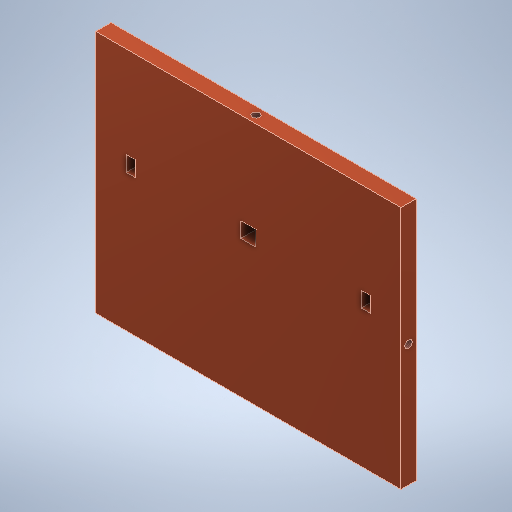
# Autodesk Inventor part: chassis arriere
Saved by Autodesk Inventor 2026.2 (Build 302298010, 298A)
## iProperties
Created: 2026-03-16
Part Number: chassis arriere
Material: Générique
Document SubType Name: Modeling
Designer: genon
Density: 1 g/cm^3
Appearance: Cuivre - Satiné
Author: genon
Autodesk Inventor part; units mm, degrees
ref_plane "YZ Plane" through (0, 0, 0) normal (1, 0, 0) x (0, 1, 0)
ref_plane "XZ Plane" through (0, 0, 0) normal (0, 1, 0) x (-1, 0, 0)
ref_plane "XY Plane" through (0, 0, 0) normal (0, 0, 1) x (1, 0, 0)
sketch "Esquisse1" plane through (0, 0, 0) normal (0, 0, 1) x (1, 0, 0)
  line L0 (0, 0) -> (100, 0)
  line L1 (100, 0) -> (100, 80)
  line L2 (100, 80) -> (0, 80)
  line L3 (0, 80) -> (0, 0)
  dimension "d0" = 100
  dimension "d1" = 80
  constraints: 8 end point, 2 parallel, 1 horizontal, 1 perpendicular
  measures "d0" distance of L2.end L1.end
  measures "d1" distance of L1.end L0.end
extrude "Extrusion1" add sketch "Esquisse1" against normal blind 5
sketch "Esquisse3" plane through (100, 0, 0) normal (1, 0, 0) x (0, 0, -1)
  line L0 (0, 0) -> (0, 80) projected
  line L1 (0, 80) -> (0, 40)
  line L2 (0, 40) -> (2.5, 40)
  line L3 (0, 40) -> (2.5, 40) construction
  line L4 (0, 0) -> (2.5, 0)
  dimension "d4" = 40
  dimension "d5" = 2.5
  dimension "d6" = 0
  constraints: 8 end point, 3 horizontal, 1 coincident, 1 collinear, 1 midpoint
  measures "d4" distance of L0.end L1.end
  measures "d5" distance of L1.end L2.end
  measures "d6" distance between parallel lines of L2 L3
hole "Perçage1" at (100, 40, -2.5) direction (-1, 0, 0) diameter 2.459 depth 8.8 tip angle 118 thread size "M3x0.5" class "6H" standard "ISO Metric profile"
sketch "Esquisse4" plane through (0, 0, 0) normal (-1, 0, 0) x (0, 0, 1)
  line L0 (0, 0) -> (-5, 0) projected
  line L1 (0, 0) -> (0, 80) projected
  line L2 (0, 80) -> (-2.5, 80)
  line L3 (-2.5, 80) -> (-2.5, 40)
  dimension "d17" = 40
  dimension "d18" = 90
  dimension "d52" = 2.5
  constraints: 4 end point, 1 coincident, 1 horizontal, 1 perpendicular
  measures "d17" distance of L2.end L3.end
  measures "d18" angle of L3 L2
  measures "d52" distance between parallel lines of L1 L3
hole "Perçage2" at (0, 40, -2.5) direction (1, 0, 0) diameter 2.459 depth 8.8 tip angle 118 thread size "M3x0.5" class "6H" standard "ISO Metric profile"
sketch "Esquisse5" plane through (0, 80, 0) normal (0, 1, 0) x (1, 0, 0)
  line L0 (100, 0) -> (0, 0) projected
  line L1 (100, 5) -> (0, 5) projected
  line L2 (0, 0) -> (0, 2.5)
  line L3 (0, 0) -> (0, 5) projected
  line L4 (0, 2.5) -> (50, 2.5)
  point P0 (50, 2.5)
  dimension "d41" = 50
  constraints: 4 end point, 1 coincident, 1 midpoint, 1 perpendicular
  measures "d41" distance of L2.end L4.end
hole "Perçage3" at (50, 80, -2.5) direction (0, -1, 0) diameter 2.459 depth 8.8 tip angle 118 thread size "M3x0.5" class "6H" standard "ISO Metric profile"
sketch "Esquisse6" plane through (0, 0, 0) normal (0, -1, 0) x (1, 0, 0)
  line L0 (0, 0) -> (100, 0) projected
  line L1 (0, -5) -> (100, -5) projected
  line L2 (0, 0) -> (0, -2.5)
  line L3 (0, -2.5) -> (50, -2.5)
  point P0 (50, -2.5)
  dimension "d40" = 50
  constraints: 4 end point, 1 coincident, 1 perpendicular, 1 vertical
  measures "d40" distance of L2.end L3.end
hole "Perçage4" at (50, 0, -2.5) direction (0, 1, 0) diameter 2.459 depth 8.8 tip angle 118 thread size "M3x0.5" class "6H" standard "ISO Metric profile"
sketch "Esquisse7" plane through (0, 0, 0) normal (0, 0, 1) x (1, 0, 0)
  line L0 (0, 0) -> (0, 45)
  line L1 (0, 0) -> (0, 80) projected
  line L2 (0, 45) -> (100, 45)
  line L3 (50, 45) -> (10, 45)
  line L4 (50, 45) -> (90, 45)
  line L5 (10, 45) -> (13, 45)
  line L6 (13, 45) -> (13, 50)
  line L7 (13, 50) -> (10, 50)
  line L8 (10, 50) -> (10, 45)
  line L9 (90, 45) -> (87, 45)
  line L10 (87, 45) -> (87, 50)
  line L11 (87, 50) -> (90, 50)
  line L12 (90, 50) -> (90, 45)
  line L13 (50, 45) -> (52.5, 45)
  line L14 (52.5, 45) -> (52.5, 50)
  line L15 (52.5, 50) -> (47.5, 50)
  line L16 (47.5, 50) -> (47.5, 45)
  line L17 (50, 45) -> (47.5, 45)
  dimension "d42" = 45
  dimension "d43" = 100
  dimension "d44" = 40
  dimension "d45" = 40
  dimension "d46" = 3
  dimension "d47" = 5
  dimension "d48" = 3
  dimension "d49" = 5
  dimension "d53" = 2.5
  dimension "d54" = 5
  dimension "d55" = 5
  constraints: 34 end point, 6 perpendicular, 5 point on line, 4 parallel, 2 horizontal, 1 collinear, 1 midpoint
  measures "d42" distance of L0.start L0.end
  measures "d43" distance of L0.end L2.end
  measures "d44" distance of L3.start L3.end
  measures "d45" distance of L3.start L4.end
  measures "d46" distance of L7.end L6.end
  measures "d47" distance of L6.end L5.end
  measures "d48" distance of L10.end L11.end
  measures "d49" distance of L9.end L10.end
  measures "d53" distance of L3.start L13.end
  measures "d54" distance of L13.end L14.end
  measures "d55" distance of L14.end L15.end
extrude "Extrusion2" cut sketch "Esquisse7" against normal through all
